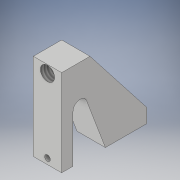
# Autodesk Inventor part: Hole part
Saved by Autodesk Inventor 2017.1 (Build 211199000, 199)
## iProperties
Created: 2017-05-02
Part Number: Hole part
Material: Generic
Document SubType Name: Modeling
Designer: 196918
Density: 1 g/cm^3
Appearance: Default
Author: 196918
Autodesk Inventor part; units mm, degrees
ref_plane "YZ Plane" through (0, 0, 0) normal (1, 0, 0) x (0, 1, 0)
ref_plane "XZ Plane" through (0, 0, 0) normal (0, 1, 0) x (-1, 0, 0)
ref_plane "XY Plane" through (0, 0, 0) normal (0, 0, 1) x (1, 0, 0)
sketch "Sketch1" plane through (0, 0, 0) normal (1, 0, 0) x (0, 1, 0)
  point P0 (0, 0)
sketch "Sketch2" plane through (0, 0, 0) normal (1, 0, 0) x (0, 1, 0)
  line L0 (29.0822, 42.9634) -> (29.0822, 36.776)
  line L1 (29.0822, 36.776) -> (-3.4283, 11.376)
  line L2 (-3.4283, 11.376) -> (-9.7783, 11.376)
  line L3 (-9.7783, 11.376) -> (-9.7783, 29.8843)
  line L4 (-9.7783, 29.8843) -> (13.0817, 38.4937)
  line L5 (10.2262, 44.396) -> (-9.7798, 44.396)
  line L6 (-9.7798, 44.396) -> (-9.7798, 49.476)
  line L7 (-9.7798, 49.476) -> (29.0822, 49.476)
  line L8 (29.0822, 49.476) -> (29.0822, 42.9634)
  line L9 (10.2262, 44.396) -> (11.4561, 44.396)
  arc A0 (13.0817, 38.4937) -> (11.4561, 44.396) centre (11.4561, 41.221) ccw
  point P0 (0, 0)
  dimension "d0" = 5.08
  dimension "d1" = 6.35
  dimension "d2" = 38.1
  dimension "d3" = 38
  dimension "d4" = 3.175
  dimension "d5" = 21.2344
  dimension "d6" = 12.7
  dimension "d7" = 38.862
  dimension "d9" = 22.86
  constraints: 20 end point, 4 perpendicular, 2 horizontal, 2 point on circle, 1 centre point, 1 collinear, 1 tangent, 1 vertical
  measures "d0" distance of L5.end L6.end
  measures "d1" distance of L1.end L2.end
  measures "d2" distance between parallel lines of L2 L7
  measures "d3" angle of L1 L7
  measures "d4" radius of A0
  measures "d5" distance from line of L3 A0.centre
  measures "d6" distance of L0.end L7.end
  measures "d7" distance of L6.end L7.end
  measures "d9" horizontal distance of L3.end L4.end
extrude "Extrusion1" add sketch "Sketch2" along normal blind 12.7
sketch "Sketch4" plane through (0, -9.7798, 49.476) normal (0, 0, 1) x (1, 0, 0)
  point P0 (0, 9.7798)
  point P1 (6.35, 35.3841)
hole "Hole1" at (6.35, 25.6044, 49.476) direction (0, 0, -1) diameter 6.4008 depth 7.62 tip angle 118 thread size "5/16-18 UNC" class "2B" standard "ANSI Unified Screw Threads"
sketch "Sketch5" plane through (0, -9.7798, 49.476) normal (0, 0, 1) x (1, 0, 0)
  point P0 (0, 9.7798)
  point P1 (6.35, 2.5513)
hole "Hole2" at (6.35, -7.2284, 49.476) direction (0, 0, -1) diameter 2.54 depth 4.445 tip angle 118
sketch "Sketch6" plane through (12.7, 29.0822, 36.776) normal (0, 0.6157, -0.788) x (-1, 0, 0)
  line L0 (12.7, -46.2603) -> (0, -46.2603) construction
  line L1 (6.35, -46.2603) -> (6.35, -0.205) construction
  line L2 (12.7, 0) -> (0, 0) construction
  point P0 (12.7, -45.5586)
  point P1 (6.35, -8.5344)
  point P2 (6.35, -18.6944)
  point P3 (6.35, -30.1244)
  point P4 (6.35, -38.1)
  dimension "d26" = 8.5344
  dimension "d27" = 18.6944
  dimension "d28" = 30.1244
  dimension "d29" = 38.1
  constraints: 4 point on line, 2 end point, 1 midpoint, 1 vertical
  measures "d26" distance from line of L2 point (6.35, -8.534)
  measures "d27" distance from line of L2 point (6.35, -18.694)
  measures "d28" distance from line of L2 point (6.35, -30.124)
  measures "d29" distance from line of L2 point (6.35, -38.1)
hole "Hole3" at (6.35, 22.357, 31.5217) at (6.35, 14.3508, 25.2665) at (6.35, 5.3439, 18.2295) at (6.35, -0.941, 13.3193) direction (0, -0.6157, 0.788) diameter 5.7404 depth 10.16 tip angle 118
body "Solid1"
